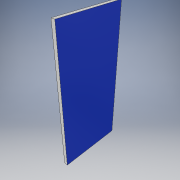
# Autodesk Inventor part: VoltageCionvertor
Saved by Autodesk Inventor 2018 (Build 220112000, 112)
## iProperties
Created: 2018-09-18
Part Number: VoltageCionvertor
Material: Generic
Document SubType Name: Modeling
Designer: Viraj Shah
Density: 1 g/cm^3
Appearance: Default
Author: Viraj Shah
Autodesk Inventor part; units mm, degrees
ref_plane "YZ Plane" through (0, 0, 0) normal (1, 0, 0) x (0, 1, 0)
ref_plane "XZ Plane" through (0, 0, 0) normal (0, 1, 0) x (-1, 0, 0)
ref_plane "XY Plane" through (0, 0, 0) normal (0, 0, 1) x (1, 0, 0)
sketch "Sketch1" plane through (0, 0, 0) normal (1, 0, 0) x (0, 1, 0)
  line L0 (-8.6, 18.65) -> (8.6, 18.65)
  line L1 (8.6, 18.65) -> (8.6, -18.65)
  line L2 (8.6, -18.65) -> (-8.6, -18.65)
  line L3 (-8.6, -18.65) -> (-8.6, 18.65)
  line L4 (-8.6, 18.65) -> (8.6, -18.65) construction
  line L5 (8.6, 18.65) -> (-8.6, -18.65) construction
  point P0 (0, 0)
  dimension "d0" = 17.2
  dimension "d1" = 37.3
  constraints: 12 end point, 2 midpoint, 2 parallel, 1 horizontal, 1 perpendicular
  measures "d0" distance of L1.end L2.end
  measures "d1" distance of L0.end L1.end
extrude "Extrusion1" add sketch "Sketch1" along normal blind 1
body "Solid1"
